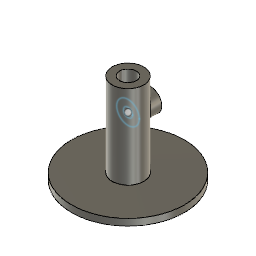
servo-pushers (Autodesk Fusion 360 design; units mm, degrees)
part number: 2026-01-12-14-36-56-861
Autodesk Fusion 360 part; units mm, degrees
note: some values were not read from the file. Set by a fixed rule: which sketch regions a step uses.
sketch "Sketch1" plane through (0, 0, 0) normal (0, 0, 1) x (1, 0, 0)
  circle A0 centre (0, 0) radius 12.5
  circle A1 centre (0, 0) radius 3.5
  dimension "d1" = 25
  dimension "d3" = 7
  constraint coincident A0.centre A1.centre
  constraint concentric A0 A1
  measures "d1" diameter of A0
  measures "d3" diameter of A1
extrude "Extrude9" add sketch "Sketch1" along normal blind 1.5 contours A0 | A1
extrude "Extrude10" add sketch "Sketch1" along normal blind 20 contours A1
sketch "Sketch3" plane through (0, 0, 20) normal (0, 0, 1) x (-1, 0, 0)
  circle A0 centre (0, 0) radius 3.5
  circle A1 centre (0, 0) radius 1.85
  dimension "d26" = 3.7
  constraint coincident A0.centre A1.centre
  measures "d26" diameter of A1
extrude "Extrude11" cut sketch "Sketch3" against normal blind 15 contours A1
sketch "Sketch4" plane through (0, 0, 0) normal (0, 1, 0) x (1, 0, 0)
  circle A0 centre (0, -13) radius 1
  circle A1 centre (0, -13) radius 2.5
  dimension "d29" = 2
  dimension "d30" = 5
  constraint concentric A0 A1
  measures "d29" diameter of A0
  measures "d30" diameter of A1
extrude "Extrude12" add sketch "Sketch4" along normal blind 5
extrude "Extrude13" cut sketch "Sketch3" against normal blind 15 contours A1
extrude "Extrude14" cut sketch "Sketch4" along normal blind 7 contours A0
sketch "Sketch2" plane through (0, 0, 0) normal (1, 0, 0) x (0, 1, 0)
  circle A0 centre (0, 6) radius 1
  circle A1 centre (0, 6) radius 2
  dimension "d14" = 2
  dimension "d15" = 4
  constraint concentric A0 A1
  measures "d14" diameter of A0
  measures "d15" diameter of A1
extrude "Extrude7" [suppressed]
extrude "Extrude8" [suppressed]
extrude "Extrude1" [suppressed]
extrude "Extrude2" [suppressed]
extrude "Extrude3" [suppressed]
